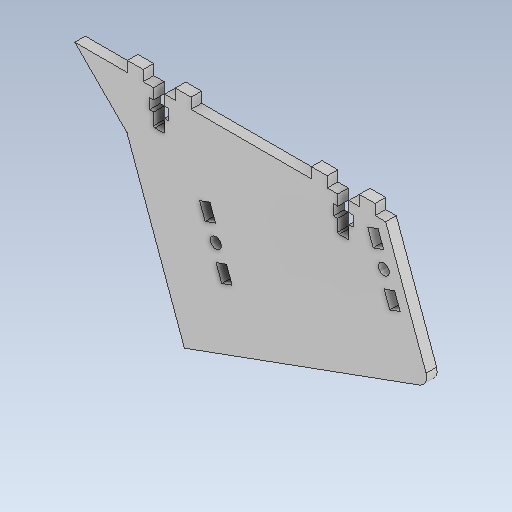
# Autodesk Inventor part: tc_support_front
Saved by Autodesk Inventor 2020.1 (Build 241239000, 239)
## iProperties
Created: 2019-07-16
Part Number: tc_support_front
Material: Acier inoxydable
Document SubType Name: Modeling
Designer: Thibault
Density: 8 g/cm^3
Appearance: Semi-poli
Author: Thibault
Autodesk Inventor part; units mm, degrees
ref_plane "YZ Plane" through (0, 0, 0) normal (1, 0, 0) x (0, 1, 0)
ref_plane "XZ Plane" through (0, 0, 0) normal (0, 1, 0) x (-1, 0, 0)
ref_plane "XY Plane" through (0, 0, 0) normal (0, 0, 1) x (1, 0, 0)
sketch "Anchor (screw side)" plane through (0, 0, 0) normal (0, 0, 1) x (1, 0, 0)
  circle A0 centre (93.8994, 50.3042) radius 1.05
  line L0 (90.8494, 51.3542) -> (87.7494, 51.3542)
  line L1 (87.7494, 51.3542) -> (87.7494, 49.2542)
  line L2 (87.7494, 49.2542) -> (90.8494, 49.2542)
  line L3 (90.8494, 49.2542) -> (90.8494, 51.3542)
  line L4 (100.0494, 51.3542) -> (96.9494, 51.3542)
  line L5 (96.9494, 51.3542) -> (96.9494, 49.2542)
  line L6 (96.9494, 49.2542) -> (100.0494, 49.2542)
  line L7 (100.0494, 49.2542) -> (100.0494, 51.3542)
  line L8 (90.8494, 51.3542) -> (96.9494, 49.2542) construction
  line L9 (96.9494, 51.3542) -> (90.8494, 49.2542) construction
  line L10 (85.7494, 53.3542) -> (102.0494, 53.3542) construction
  line L11 (102.0494, 53.3542) -> (102.0494, 47.2542) construction
  line L12 (102.0494, 47.2542) -> (85.7494, 47.2542) construction
  line L13 (85.7494, 47.2542) -> (85.7494, 53.3542) construction
  point P0 (103.5798, 50.1132)
  dimension "d27" = 2.1
  dimension "d28" = 3.1
  dimension "d29" = 2.1
  dimension "slot_distance" = 6.1
  dimension "d34" = 2
  dimension "d35_1" = 2
  dimension "d36_1" = 2
  dimension "d37" = 2
  measures "d27" diameter of A0
  measures "d28" distance of L2.end L1.end
  measures "d29" distance of L1.end L0.end
  measures "slot_distance" distance between parallel lines of L5 L3
  measures "d34" distance between parallel lines of L0 L10
  measures "d35_1" distance between parallel lines of L12 L2
  measures "d36_1" distance between parallel lines of L11 L7
  measures "d37" distance between parallel lines of L13 L1
sketch "Anchor (nut side)" plane through (0, 0, 0) normal (0, 0, 1) x (1, 0, 0)
  line L0 (11.1, 0) -> (9.1, 0)
  line L1 (9.1, 0) -> (9.1, -2)
  line L2 (9.1, -2) -> (9.9, -2)
  line L3 (9.9, -2) -> (9.9, -4)
  line L4 (6.2, -4) -> (6.2, -2)
  line L5 (6.2, -2) -> (7, -2)
  line L6 (7, -2) -> (7, 0)
  line L7 (7, 0) -> (5, 0)
  line L8 (2, 0) -> (2, 2)
  line L9 (2, 0) -> (3, 0) construction
  line L10 (2, 2) -> (5, 2)
  line L11 (5, 2) -> (5, 0)
  line L12 (11.1, 0) -> (11.1, 2)
  line L13 (11.1, 2) -> (14.1, 2)
  line L14 (14.1, 2) -> (14.1, 0)
  line L15 (0, 0) -> (2, 0)
  line L16 (14.1, 0) -> (16.1, 0)
  line L17 (6.2, -4) -> (7, -4)
  line L18 (9.9, -4) -> (9.1, -4)
  line L19 (7, -4) -> (7, -6.25)
  line L20 (9.1, -4) -> (9.1, -6.25)
  line L21 (7.25, -6.5) -> (8.05, -6.5)
  arc A0 (7, -6.25) -> (7.25, -6.5) centre (7.25, -6.25) ccw
  arc A1 (8.85, -6.5) -> (9.1, -6.25) centre (8.85, -6.25) ccw
  line L22 (8.05, -6.5) -> (8.85, -6.5)
  line L23 (8.05, -3.8983) -> (8.05, -9.959) construction
  point P0 (9.1321, -0.6227)
  point P1 (7, -6.5)
  point P2 (9.1, -6.5)
  dimension "d3" = 2
  dimension "d7" = 6.1
  dimension "d10" = 2
  dimension "d11" = 2
  dimension "d12" = 0.8
  dimension "d13" = 2
  dimension "d14" = 0.8
  dimension "d15" = 2.1
  dimension "d18" = 2
  dimension "d19" = 0.8
  dimension "d20" = 0.8
  dimension "d21" = 2.5
  dimension "d22" = 2.5
  dimension "d23" = 2.1
  dimension "d38" = 2
  dimension "d39" = 0.25
  dimension "d120" = 3
  measures "d3" distance of L15.start L8.start
  measures "d7" distance of L7.end L0.start
  measures "d10" distance of L0.start L0.end
  measures "d11" distance of L0.end L1.end
  measures "d12" distance of L1.end L2.end
  measures "d13" distance of L2.end L3.end
  measures "d14" distance of L4.end L5.end
  measures "d15" distance of L6.end L0.end
  measures "d18" distance of L14.end L16.end
  measures "d19" distance of L4.start L17.end
  measures "d20" distance of L3.end L18.end
  measures "d21" distance of L17.end point (7, -6.5)
  measures "d22" distance of L18.end point (9.1, -6.5)
  measures "d23" distance of L17.end L18.end
  measures "d38" distance between parallel lines of L15 L10
  measures "d39" radius of A0
  measures "d120" distance of L8.end L10.end
derived "shared_parameters.ipt"
sketch "Esquisse1" plane through (0, 0, 0) normal (0, 0, 1) x (1, 0, 0)
  line L0 (-12.2169, 6.8501) -> (6.6831, 6.8501)
  line L1 (-28.3169, 6.8501) -> (-36.3169, 6.8501)
  line L2 (-36.3169, 6.8501) -> (-26.4133, -3.0535)
  line L3 (30.4625, -14.2491) -> (22.7831, 6.8501)
  line L4 (29.2672, -16.8125) -> (-15.4779, -33.0984)
  line L5 (-2.0657, -1.8526) -> (7.9343, -1.7975) construction
  arc A0 (29.2672, -16.8125) -> (30.4625, -14.2491) centre (28.5832, -14.9331) ccw
  line L6 (-15.4779, -33.0984) -> (-26.4133, -3.0535)
  line L7 (-17.2169, 6.8501) -> (-19.2169, 6.8501)
  line L8 (-19.2169, 6.8501) -> (-19.2169, 4.8501)
  line L9 (-19.2169, 4.8501) -> (-18.4169, 4.8501)
  line L10 (-18.4169, 4.8501) -> (-18.4169, 2.8501)
  line L11 (-22.1169, 2.8501) -> (-22.1169, 4.8501)
  line L12 (-22.1169, 4.8501) -> (-21.3169, 4.8501)
  line L13 (-21.3169, 4.8501) -> (-21.3169, 6.8501)
  line L14 (-21.3169, 6.8501) -> (-23.3169, 6.8501)
  line L15 (-26.3169, 6.8501) -> (-26.3169, 8.8501)
  line L16 (-26.3169, 6.8501) -> (-25.3169, 6.8501) construction
  line L17 (-26.3169, 8.8501) -> (-23.3169, 8.8501)
  line L18 (-23.3169, 8.8501) -> (-23.3169, 6.8501)
  line L19 (-17.2169, 6.8501) -> (-17.2169, 8.8501)
  line L20 (-17.2169, 8.8501) -> (-14.2169, 8.8501)
  line L21 (-14.2169, 8.8501) -> (-14.2169, 6.8501)
  line L22 (-28.3169, 6.8501) -> (-26.3169, 6.8501)
  line L23 (-14.2169, 6.8501) -> (-12.2169, 6.8501)
  line L24 (-22.1169, 2.8501) -> (-21.3169, 2.8501)
  line L25 (-18.4169, 2.8501) -> (-19.2169, 2.8501)
  line L26 (-21.3169, 2.8501) -> (-21.3169, 0.6001)
  line L27 (-19.2169, 2.8501) -> (-19.2169, 0.6001)
  line L28 (-21.0669, 0.3501) -> (-20.2669, 0.3501)
  arc A1 (-21.3169, 0.6001) -> (-21.0669, 0.3501) centre (-21.0669, 0.6001) ccw
  arc A2 (-19.4669, 0.3501) -> (-19.2169, 0.6001) centre (-19.4669, 0.6001) ccw
  line L29 (-20.2669, 0.3501) -> (-19.4669, 0.3501)
  line L30 (-20.2669, 2.9518) -> (-20.2669, -3.1089) construction
  line L31 (17.7831, 6.8501) -> (15.7831, 6.8501)
  line L32 (15.7831, 6.8501) -> (15.7831, 4.8501)
  line L33 (15.7831, 4.8501) -> (16.5831, 4.8501)
  line L34 (16.5831, 4.8501) -> (16.5831, 2.8501)
  line L35 (12.8831, 2.8501) -> (12.8831, 4.8501)
  line L36 (12.8831, 4.8501) -> (13.6831, 4.8501)
  line L37 (13.6831, 4.8501) -> (13.6831, 6.8501)
  line L38 (13.6831, 6.8501) -> (11.6831, 6.8501)
  line L39 (8.6831, 6.8501) -> (8.6831, 8.8501)
  line L40 (8.6831, 6.8501) -> (9.6831, 6.8501) construction
  line L41 (8.6831, 8.8501) -> (11.6831, 8.8501)
  line L42 (11.6831, 8.8501) -> (11.6831, 6.8501)
  line L43 (17.7831, 6.8501) -> (17.7831, 8.8501)
  line L44 (17.7831, 8.8501) -> (20.7831, 8.8501)
  line L45 (20.7831, 8.8501) -> (20.7831, 6.8501)
  line L46 (6.6831, 6.8501) -> (8.6831, 6.8501)
  line L47 (20.7831, 6.8501) -> (22.7831, 6.8501)
  line L48 (12.8831, 2.8501) -> (13.6831, 2.8501)
  line L49 (16.5831, 2.8501) -> (15.7831, 2.8501)
  line L50 (13.6831, 2.8501) -> (13.6831, 0.6001)
  line L51 (15.7831, 2.8501) -> (15.7831, 0.6001)
  line L52 (13.9331, 0.3501) -> (14.7331, 0.3501)
  arc A3 (13.6831, 0.6001) -> (13.9331, 0.3501) centre (13.9331, 0.6001) ccw
  arc A4 (15.5331, 0.3501) -> (15.7831, 0.6001) centre (15.5331, 0.6001) ccw
  line L53 (14.7331, 0.3501) -> (15.5331, 0.3501)
  line L54 (14.7331, 2.9518) -> (14.7331, -3.1089) construction
  circle A5 centre (22.4491, -1.1499) radius 1.05
  line L55 (22.5056, -4.3751) -> (23.5658, -7.2881)
  line L56 (23.5658, -7.2881) -> (25.5392, -6.5699)
  line L57 (25.5392, -6.5699) -> (24.4789, -3.6568)
  line L58 (24.4789, -3.6568) -> (22.5056, -4.3751)
  line L59 (19.359, 4.2701) -> (20.4192, 1.357)
  line L60 (20.4192, 1.357) -> (22.3926, 2.0753)
  line L61 (22.3926, 2.0753) -> (21.3323, 4.9883)
  line L62 (21.3323, 4.9883) -> (19.359, 4.2701)
  line L63 (22.5056, -4.3751) -> (22.3926, 2.0753) construction
  line L64 (20.4192, 1.357) -> (24.4789, -3.6568) construction
  line L65 (22.3705, -9.8515) -> (16.7956, 5.4654) construction
  line L66 (16.7956, 5.4654) -> (22.5277, 7.5518) construction
  line L67 (22.5277, 7.5518) -> (28.1026, -7.7652) construction
  line L68 (28.1026, -7.7652) -> (22.3705, -9.8515) construction
  circle A6 centre (-9.5005, -12.7786) radius 1.05
  line L69 (-9.557, -9.5534) -> (-10.6172, -6.6403)
  line L70 (-10.6172, -6.6403) -> (-12.5906, -7.3586)
  line L71 (-12.5906, -7.3586) -> (-11.5303, -10.2716)
  line L72 (-11.5303, -10.2716) -> (-9.557, -9.5534)
  line L73 (-6.4104, -18.1986) -> (-7.4706, -15.2855)
  line L74 (-7.4706, -15.2855) -> (-9.444, -16.0038)
  line L75 (-9.444, -16.0038) -> (-8.3837, -18.9168)
  line L76 (-8.3837, -18.9168) -> (-6.4104, -18.1986)
  line L77 (-9.557, -9.5534) -> (-9.444, -16.0038) construction
  line L78 (-7.4706, -15.2855) -> (-11.5303, -10.2716) construction
  line L79 (-9.4219, -4.0769) -> (-3.8469, -19.3939) construction
  line L80 (-3.8469, -19.3939) -> (-9.5791, -21.4802) construction
  line L81 (-9.5791, -21.4802) -> (-15.154, -6.1632) construction
  line L82 (-15.154, -6.1632) -> (-9.4219, -4.0769) construction
  point P0 (31.1466, -16.1285)
  point P1 (22.4992, -2.0098)
  point P2 (22.4491, -1.1499)
  point P3 (-9.5005, -12.7786)
  point P4 (22.7831, 6.8501)
  dimension "d33" = 59.1
  dimension "d44" = 10.9
  dimension "d46" = 2
  dimension "d49" = 10
  dimension "d52" = 2
  dimension "d53" = 36
  dimension "d54" = 8
  dimension "d57" = 45
  dimension "d58" = 20
  constraints: 14 end point, 3 horizontal, 2 point on circle, 2 point on line, 2 tangent, 1 centre point, 1 parallel, 1 perpendicular, 6 other
  measures "d33" distance of L3.end L1.end
  measures "d46" radius of A0
  measures "d57" angle of L2 L1
  measures "d58" angle of L4 L0
extrude "Extrusion1" add sketch "Esquisse1" along normal blind 2
derived "tc_base_plate.ipt"
equation "\"d33\" = tc_base_width"
equation "\"d44\" = extra_height_front"
equation "\"d52\" = anchor_dist_a"
equation "\"d53\" = anchor_dist_b"
equation "\"d54\" = anchor_dist_top_a"
equation "\"d58\" = tilt_angle"
equation "\"d35\" = sheet_thickness"
equation "\"tc_base_width\" = 59.1"
equation "\"extra_height_front\" = 10.9"
equation "\"anchor_dist_a\" = 2"
equation "\"anchor_dist_b\" = 36"
equation "\"anchor_dist_top_a\" = 8"
equation "\"tilt_angle\" = 20deg"
equation "\"sheet_thickness\" = 2"
